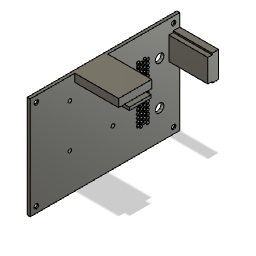
Main Pi Lid v6 (Autodesk Fusion 360 design; units mm, degrees)
Autodesk Fusion 360 part; units mm, degrees
sketch "Sketch1" plane through (0, 0, 0) normal (1, 0, 0) x (0, 0, -1)
  line L0 (-52, 35.5) -> (52, 35.5)
  line L1 (52, 35.5) -> (52, -35.5)
  line L2 (52, -35.5) -> (-52, -35.5)
  line L3 (-52, -35.5) -> (-52, 35.5)
  line L4 (-52, 35.5) -> (52, -35.5) construction
  line L5 (52, 35.5) -> (-52, -35.5) construction
  circle A0 centre (-47.75, 31.25) radius 1.55
  circle A1 centre (47.75, 31.25) radius 1.55
  circle A2 centre (47.75, -31.25) radius 1.55
  circle A3 centre (-47.75, -31.25) radius 1.55
  line L6 (20.5, 35.5) -> (-39.5, 35.5)
  line L7 (-39.5, 35.5) -> (-39.5, -24.5)
  line L8 (-39.5, -24.5) -> (20.5, -24.5)
  line L9 (20.5, -24.5) -> (20.5, 35.5)
  line L10 (20.5, 35.5) -> (-39.5, -24.5) construction
  line L11 (-39.5, 35.5) -> (20.5, -24.5) construction
  circle A4 centre (5.5, 20.5) radius 1.25
  circle A5 centre (-24.5, 20.5) radius 1.25
  circle A6 centre (-24.5, -9.5) radius 1.25
  circle A7 centre (5.5, -9.5) radius 1.25
  circle A8 centre (38, 15) radius 3
  circle A9 centre (38, -15) radius 3
  line L12 (22.4227, 20.645) -> (21.8453, 19.645)
  line L13 (21.8453, 19.645) -> (22.4227, 18.645)
  line L14 (22.4227, 18.645) -> (23.5774, 18.645)
  line L15 (23.5774, 18.645) -> (24.1547, 19.645)
  line L16 (24.1547, 19.645) -> (23.5774, 20.645)
  line L17 (23.5774, 20.645) -> (22.4227, 20.645)
  line L18 (24.653, 19.3561) -> (24.0756, 18.3561)
  line L19 (24.0756, 18.3561) -> (24.653, 17.3561)
  line L20 (24.653, 17.3561) -> (25.8077, 17.3561)
  line L21 (25.8077, 17.3561) -> (26.385, 18.3561)
  line L22 (26.385, 18.3561) -> (25.8077, 19.3561)
  line L23 (25.8077, 19.3561) -> (24.653, 19.3561)
  line L24 (30.3077, 19.3561) -> (29.153, 19.3561)
  line L25 (26.3453, 19.645) -> (26.9227, 18.645)
  line L26 (26.9227, 18.645) -> (28.0774, 18.645)
  line L27 (29.153, 19.3561) -> (28.5756, 18.3561)
  line L28 (29.153, 17.3561) -> (30.3077, 17.3561)
  line L29 (30.3077, 17.3561) -> (30.885, 18.3561)
  line L30 (28.6547, 19.645) -> (28.0774, 20.645)
  line L31 (28.5756, 18.3561) -> (29.153, 17.3561)
  line L32 (28.0774, 20.645) -> (26.9227, 20.645)
  line L33 (30.885, 18.3561) -> (30.3077, 19.3561)
  line L34 (28.0774, 18.645) -> (28.6547, 19.645)
  line L35 (26.9227, 20.645) -> (26.3453, 19.645)
  line L36 (25.8077, 16.8228) -> (24.653, 16.8228)
  line L37 (21.8453, 17.1117) -> (22.4227, 16.1117)
  line L38 (22.4227, 16.1117) -> (23.5774, 16.1117)
  line L39 (24.653, 16.8228) -> (24.0756, 15.8228)
  line L40 (24.653, 14.8228) -> (25.8077, 14.8228)
  line L41 (25.8077, 14.8228) -> (26.385, 15.8228)
  line L42 (24.1547, 17.1117) -> (23.5774, 18.1117)
  line L43 (24.0756, 15.8228) -> (24.653, 14.8228)
  line L44 (23.5774, 18.1117) -> (22.4227, 18.1117)
  line L45 (26.385, 15.8228) -> (25.8077, 16.8228)
  line L46 (23.5774, 16.1117) -> (24.1547, 17.1117)
  line L47 (22.4227, 18.1117) -> (21.8453, 17.1117)
  line L48 (30.3077, 16.8228) -> (29.153, 16.8228)
  line L49 (26.3453, 17.1117) -> (26.9227, 16.1117)
  line L50 (26.9227, 16.1117) -> (28.0774, 16.1117)
  line L51 (29.153, 16.8228) -> (28.5756, 15.8228)
  line L52 (29.153, 14.8228) -> (30.3077, 14.8228)
  line L53 (30.3077, 14.8228) -> (30.885, 15.8228)
  line L54 (28.6547, 17.1117) -> (28.0774, 18.1117)
  line L55 (28.5756, 15.8228) -> (29.153, 14.8228)
  line L56 (28.0774, 18.1117) -> (26.9227, 18.1117)
  line L57 (30.885, 15.8228) -> (30.3077, 16.8228)
  line L58 (28.0774, 16.1117) -> (28.6547, 17.1117)
  line L59 (26.9227, 18.1117) -> (26.3453, 17.1117)
  line L60 (25.8077, 14.2895) -> (24.653, 14.2895)
  line L61 (21.8453, 14.5783) -> (22.4227, 13.5783)
  line L62 (22.4227, 13.5783) -> (23.5774, 13.5783)
  line L63 (24.653, 14.2895) -> (24.0756, 13.2895)
  line L64 (24.653, 12.2895) -> (25.8077, 12.2895)
  line L65 (25.8077, 12.2895) -> (26.385, 13.2895)
  line L66 (24.1547, 14.5783) -> (23.5774, 15.5783)
  line L67 (24.0756, 13.2895) -> (24.653, 12.2895)
  line L68 (23.5774, 15.5783) -> (22.4227, 15.5783)
  line L69 (26.385, 13.2895) -> (25.8077, 14.2895)
  line L70 (23.5774, 13.5783) -> (24.1547, 14.5783)
  line L71 (22.4227, 15.5783) -> (21.8453, 14.5783)
  line L72 (30.3077, 14.2895) -> (29.153, 14.2895)
  line L73 (26.3453, 14.5783) -> (26.9227, 13.5783)
  line L74 (26.9227, 13.5783) -> (28.0774, 13.5783)
  line L75 (29.153, 14.2895) -> (28.5756, 13.2895)
  line L76 (29.153, 12.2895) -> (30.3077, 12.2895)
  line L77 (30.3077, 12.2895) -> (30.885, 13.2895)
  line L78 (28.6547, 14.5783) -> (28.0774, 15.5783)
  line L79 (28.5756, 13.2895) -> (29.153, 12.2895)
  line L80 (28.0774, 15.5783) -> (26.9227, 15.5783)
  line L81 (30.885, 13.2895) -> (30.3077, 14.2895)
  line L82 (28.0774, 13.5783) -> (28.6547, 14.5783)
  line L83 (26.9227, 15.5783) -> (26.3453, 14.5783)
  line L84 (25.8077, 11.7561) -> (24.653, 11.7561)
  line L85 (21.8453, 12.045) -> (22.4227, 11.045)
  line L86 (22.4227, 11.045) -> (23.5774, 11.045)
  line L87 (24.653, 11.7561) -> (24.0756, 10.7561)
  line L88 (24.653, 9.7561) -> (25.8077, 9.7561)
  line L89 (25.8077, 9.7561) -> (26.385, 10.7561)
  line L90 (24.1547, 12.045) -> (23.5774, 13.045)
  line L91 (24.0756, 10.7561) -> (24.653, 9.7561)
  line L92 (23.5774, 13.045) -> (22.4227, 13.045)
  line L93 (26.385, 10.7561) -> (25.8077, 11.7561)
  line L94 (23.5774, 11.045) -> (24.1547, 12.045)
  line L95 (22.4227, 13.045) -> (21.8453, 12.045)
  line L96 (30.3077, 11.7561) -> (29.153, 11.7561)
  line L97 (26.3453, 12.045) -> (26.9227, 11.045)
  line L98 (26.9227, 11.045) -> (28.0774, 11.045)
  line L99 (29.153, 11.7561) -> (28.5756, 10.7561)
  line L100 (29.153, 9.7561) -> (30.3077, 9.7561)
  line L101 (30.3077, 9.7561) -> (30.885, 10.7561)
  line L102 (28.6547, 12.045) -> (28.0774, 13.045)
  line L103 (28.5756, 10.7561) -> (29.153, 9.7561)
  line L104 (28.0774, 13.045) -> (26.9227, 13.045)
  line L105 (30.885, 10.7561) -> (30.3077, 11.7561)
  line L106 (28.0774, 11.045) -> (28.6547, 12.045)
  line L107 (26.9227, 13.045) -> (26.3453, 12.045)
  line L108 (25.8077, 9.2228) -> (24.653, 9.2228)
  line L109 (21.8453, 9.5117) -> (22.4227, 8.5117)
  line L110 (22.4227, 8.5117) -> (23.5774, 8.5117)
  line L111 (24.653, 9.2228) -> (24.0756, 8.2228)
  line L112 (24.653, 7.2228) -> (25.8077, 7.2228)
  line L113 (25.8077, 7.2228) -> (26.385, 8.2228)
  line L114 (24.1547, 9.5117) -> (23.5774, 10.5117)
  line L115 (24.0756, 8.2228) -> (24.653, 7.2228)
  line L116 (23.5774, 10.5117) -> (22.4227, 10.5117)
  line L117 (26.385, 8.2228) -> (25.8077, 9.2228)
  line L118 (23.5774, 8.5117) -> (24.1547, 9.5117)
  line L119 (22.4227, 10.5117) -> (21.8453, 9.5117)
  line L120 (30.3077, 9.2228) -> (29.153, 9.2228)
  line L121 (26.3453, 9.5117) -> (26.9227, 8.5117)
  line L122 (26.9227, 8.5117) -> (28.0774, 8.5117)
  line L123 (29.153, 9.2228) -> (28.5756, 8.2228)
  line L124 (29.153, 7.2228) -> (30.3077, 7.2228)
  line L125 (30.3077, 7.2228) -> (30.885, 8.2228)
  line L126 (28.6547, 9.5117) -> (28.0774, 10.5117)
  line L127 (28.5756, 8.2228) -> (29.153, 7.2228)
  line L128 (28.0774, 10.5117) -> (26.9227, 10.5117)
  line L129 (30.885, 8.2228) -> (30.3077, 9.2228)
  line L130 (28.0774, 8.5117) -> (28.6547, 9.5117)
  line L131 (26.9227, 10.5117) -> (26.3453, 9.5117)
  line L132 (25.8077, 6.6895) -> (24.653, 6.6895)
  line L133 (21.8453, 6.9783) -> (22.4227, 5.9783)
  line L134 (22.4227, 5.9783) -> (23.5774, 5.9783)
  line L135 (24.653, 6.6895) -> (24.0756, 5.6895)
  line L136 (24.653, 4.6895) -> (25.8077, 4.6895)
  line L137 (25.8077, 4.6895) -> (26.385, 5.6895)
  line L138 (24.1547, 6.9783) -> (23.5774, 7.9783)
  line L139 (24.0756, 5.6895) -> (24.653, 4.6895)
  line L140 (23.5774, 7.9783) -> (22.4227, 7.9783)
  line L141 (26.385, 5.6895) -> (25.8077, 6.6895)
  line L142 (23.5774, 5.9783) -> (24.1547, 6.9783)
  line L143 (22.4227, 7.9783) -> (21.8453, 6.9783)
  line L144 (30.3077, 6.6895) -> (29.153, 6.6895)
  line L145 (26.3453, 6.9783) -> (26.9227, 5.9783)
  line L146 (26.9227, 5.9783) -> (28.0774, 5.9783)
  line L147 (29.153, 6.6895) -> (28.5756, 5.6895)
  line L148 (29.153, 4.6895) -> (30.3077, 4.6895)
  line L149 (30.3077, 4.6895) -> (30.885, 5.6895)
  line L150 (28.6547, 6.9783) -> (28.0774, 7.9783)
  line L151 (28.5756, 5.6895) -> (29.153, 4.6895)
  line L152 (28.0774, 7.9783) -> (26.9227, 7.9783)
  line L153 (30.885, 5.6895) -> (30.3077, 6.6895)
  line L154 (28.0774, 5.9783) -> (28.6547, 6.9783)
  line L155 (26.9227, 7.9783) -> (26.3453, 6.9783)
  line L156 (25.8077, 4.1561) -> (24.653, 4.1561)
  line L157 (21.8453, 4.445) -> (22.4227, 3.445)
  line L158 (22.4227, 3.445) -> (23.5774, 3.445)
  line L159 (24.653, 4.1561) -> (24.0756, 3.1561)
  line L160 (24.653, 2.1561) -> (25.8077, 2.1561)
  line L161 (25.8077, 2.1561) -> (26.385, 3.1561)
  line L162 (24.1547, 4.445) -> (23.5774, 5.445)
  line L163 (24.0756, 3.1561) -> (24.653, 2.1561)
  line L164 (23.5774, 5.445) -> (22.4227, 5.445)
  line L165 (26.385, 3.1561) -> (25.8077, 4.1561)
  line L166 (23.5774, 3.445) -> (24.1547, 4.445)
  line L167 (22.4227, 5.445) -> (21.8453, 4.445)
  line L168 (30.3077, 4.1561) -> (29.153, 4.1561)
  line L169 (26.3453, 4.445) -> (26.9227, 3.445)
  line L170 (26.9227, 3.445) -> (28.0774, 3.445)
  line L171 (29.153, 4.1561) -> (28.5756, 3.1561)
  line L172 (29.153, 2.1561) -> (30.3077, 2.1561)
  line L173 (30.3077, 2.1561) -> (30.885, 3.1561)
  line L174 (28.6547, 4.445) -> (28.0774, 5.445)
  line L175 (28.5756, 3.1561) -> (29.153, 2.1561)
  line L176 (28.0774, 5.445) -> (26.9227, 5.445)
  line L177 (30.885, 3.1561) -> (30.3077, 4.1561)
  line L178 (28.0774, 3.445) -> (28.6547, 4.445)
  line L179 (26.9227, 5.445) -> (26.3453, 4.445)
  line L180 (25.8077, 1.6228) -> (24.653, 1.6228)
  line L181 (21.8453, 1.9117) -> (22.4227, 0.9117)
  line L182 (22.4227, 0.9117) -> (23.5774, 0.9117)
  line L183 (24.653, 1.6228) -> (24.0756, 0.6228)
  line L184 (24.653, -0.3772) -> (25.8077, -0.3772)
  line L185 (25.8077, -0.3772) -> (26.385, 0.6228)
  line L186 (24.1547, 1.9117) -> (23.5774, 2.9117)
  line L187 (24.0756, 0.6228) -> (24.653, -0.3772)
  line L188 (23.5774, 2.9117) -> (22.4227, 2.9117)
  line L189 (26.385, 0.6228) -> (25.8077, 1.6228)
  line L190 (23.5774, 0.9117) -> (24.1547, 1.9117)
  line L191 (22.4227, 2.9117) -> (21.8453, 1.9117)
  line L192 (30.3077, 1.6228) -> (29.153, 1.6228)
  line L193 (26.3453, 1.9117) -> (26.9227, 0.9117)
  line L194 (26.9227, 0.9117) -> (28.0774, 0.9117)
  line L195 (29.153, 1.6228) -> (28.5756, 0.6228)
  line L196 (29.153, -0.3772) -> (30.3077, -0.3772)
  line L197 (30.3077, -0.3772) -> (30.885, 0.6228)
  line L198 (28.6547, 1.9117) -> (28.0774, 2.9117)
  line L199 (28.5756, 0.6228) -> (29.153, -0.3772)
  line L200 (28.0774, 2.9117) -> (26.9227, 2.9117)
  line L201 (30.885, 0.6228) -> (30.3077, 1.6228)
  line L202 (28.0774, 0.9117) -> (28.6547, 1.9117)
  line L203 (26.9227, 2.9117) -> (26.3453, 1.9117)
  line L204 (25.8077, -0.9105) -> (24.653, -0.9105)
  line L205 (21.8453, -0.6217) -> (22.4227, -1.6217)
  line L206 (22.4227, -1.6217) -> (23.5774, -1.6217)
  line L207 (24.653, -0.9105) -> (24.0756, -1.9105)
  line L208 (24.653, -2.9105) -> (25.8077, -2.9105)
  line L209 (25.8077, -2.9105) -> (26.385, -1.9105)
  line L210 (24.1547, -0.6217) -> (23.5774, 0.3783)
  line L211 (24.0756, -1.9105) -> (24.653, -2.9105)
  line L212 (23.5774, 0.3783) -> (22.4227, 0.3783)
  line L213 (26.385, -1.9105) -> (25.8077, -0.9105)
  line L214 (23.5774, -1.6217) -> (24.1547, -0.6217)
  line L215 (22.4227, 0.3783) -> (21.8453, -0.6217)
  line L216 (30.3077, -0.9105) -> (29.153, -0.9105)
  line L217 (26.3453, -0.6217) -> (26.9227, -1.6217)
  line L218 (26.9227, -1.6217) -> (28.0774, -1.6217)
  line L219 (29.153, -0.9105) -> (28.5756, -1.9105)
  line L220 (29.153, -2.9105) -> (30.3077, -2.9105)
  line L221 (30.3077, -2.9105) -> (30.885, -1.9105)
  line L222 (28.6547, -0.6217) -> (28.0774, 0.3783)
  line L223 (28.5756, -1.9105) -> (29.153, -2.9105)
  line L224 (28.0774, 0.3783) -> (26.9227, 0.3783)
  line L225 (30.885, -1.9105) -> (30.3077, -0.9105)
  line L226 (28.0774, -1.6217) -> (28.6547, -0.6217)
  line L227 (26.9227, 0.3783) -> (26.3453, -0.6217)
  line L228 (25.8077, -3.4439) -> (24.653, -3.4439)
  line L229 (21.8453, -3.155) -> (22.4227, -4.155)
  line L230 (22.4227, -4.155) -> (23.5774, -4.155)
  line L231 (24.653, -3.4439) -> (24.0756, -4.4439)
  line L232 (24.653, -5.4439) -> (25.8077, -5.4439)
  line L233 (25.8077, -5.4439) -> (26.385, -4.4439)
  line L234 (24.1547, -3.155) -> (23.5774, -2.155)
  line L235 (24.0756, -4.4439) -> (24.653, -5.4439)
  line L236 (23.5774, -2.155) -> (22.4227, -2.155)
  line L237 (26.385, -4.4439) -> (25.8077, -3.4439)
  line L238 (23.5774, -4.155) -> (24.1547, -3.155)
  line L239 (22.4227, -2.155) -> (21.8453, -3.155)
  line L240 (30.3077, -3.4439) -> (29.153, -3.4439)
  line L241 (26.3453, -3.155) -> (26.9227, -4.155)
  line L242 (26.9227, -4.155) -> (28.0774, -4.155)
  line L243 (29.153, -3.4439) -> (28.5756, -4.4439)
  line L244 (29.153, -5.4439) -> (30.3077, -5.4439)
  line L245 (30.3077, -5.4439) -> (30.885, -4.4439)
  line L246 (28.6547, -3.155) -> (28.0774, -2.155)
  line L247 (28.5756, -4.4439) -> (29.153, -5.4439)
  line L248 (28.0774, -2.155) -> (26.9227, -2.155)
  line L249 (30.885, -4.4439) -> (30.3077, -3.4439)
  line L250 (28.0774, -4.155) -> (28.6547, -3.155)
  line L251 (26.9227, -2.155) -> (26.3453, -3.155)
  line L252 (25.8077, -5.9772) -> (24.653, -5.9772)
  line L253 (21.8453, -5.6883) -> (22.4227, -6.6883)
  line L254 (22.4227, -6.6883) -> (23.5774, -6.6883)
  line L255 (24.653, -5.9772) -> (24.0756, -6.9772)
  line L256 (24.653, -7.9772) -> (25.8077, -7.9772)
  line L257 (25.8077, -7.9772) -> (26.385, -6.9772)
  line L258 (24.1547, -5.6883) -> (23.5774, -4.6883)
  line L259 (24.0756, -6.9772) -> (24.653, -7.9772)
  line L260 (23.5774, -4.6883) -> (22.4227, -4.6883)
  line L261 (26.385, -6.9772) -> (25.8077, -5.9772)
  line L262 (23.5774, -6.6883) -> (24.1547, -5.6883)
  line L263 (22.4227, -4.6883) -> (21.8453, -5.6883)
  line L264 (30.3077, -5.9772) -> (29.153, -5.9772)
  line L265 (26.3453, -5.6883) -> (26.9227, -6.6883)
  line L266 (26.9227, -6.6883) -> (28.0774, -6.6883)
  line L267 (29.153, -5.9772) -> (28.5756, -6.9772)
  line L268 (29.153, -7.9772) -> (30.3077, -7.9772)
  line L269 (30.3077, -7.9772) -> (30.885, -6.9772)
  line L270 (28.6547, -5.6883) -> (28.0774, -4.6883)
  line L271 (28.5756, -6.9772) -> (29.153, -7.9772)
  line L272 (28.0774, -4.6883) -> (26.9227, -4.6883)
  line L273 (30.885, -6.9772) -> (30.3077, -5.9772)
  line L274 (28.0774, -6.6883) -> (28.6547, -5.6883)
  line L275 (26.9227, -4.6883) -> (26.3453, -5.6883)
  line L276 (25.8077, -8.5105) -> (24.653, -8.5105)
  line L277 (21.8453, -8.2217) -> (22.4227, -9.2217)
  line L278 (22.4227, -9.2217) -> (23.5774, -9.2217)
  line L279 (24.653, -8.5105) -> (24.0756, -9.5105)
  line L280 (24.653, -10.5105) -> (25.8077, -10.5105)
  line L281 (25.8077, -10.5105) -> (26.385, -9.5105)
  line L282 (24.1547, -8.2217) -> (23.5774, -7.2217)
  line L283 (24.0756, -9.5105) -> (24.653, -10.5105)
  line L284 (23.5774, -7.2217) -> (22.4227, -7.2217)
  line L285 (26.385, -9.5105) -> (25.8077, -8.5105)
  line L286 (23.5774, -9.2217) -> (24.1547, -8.2217)
  line L287 (22.4227, -7.2217) -> (21.8453, -8.2217)
  line L288 (30.3077, -8.5105) -> (29.153, -8.5105)
  line L289 (26.3453, -8.2217) -> (26.9227, -9.2217)
  line L290 (26.9227, -9.2217) -> (28.0774, -9.2217)
  line L291 (29.153, -8.5105) -> (28.5756, -9.5105)
  line L292 (29.153, -10.5105) -> (30.3077, -10.5105)
  line L293 (30.3077, -10.5105) -> (30.885, -9.5105)
  line L294 (28.6547, -8.2217) -> (28.0774, -7.2217)
  line L295 (28.5756, -9.5105) -> (29.153, -10.5105)
  line L296 (28.0774, -7.2217) -> (26.9227, -7.2217)
  line L297 (30.885, -9.5105) -> (30.3077, -8.5105)
  line L298 (28.0774, -9.2217) -> (28.6547, -8.2217)
  line L299 (26.9227, -7.2217) -> (26.3453, -8.2217)
  line L300 (25.8077, -11.0439) -> (24.653, -11.0439)
  line L301 (21.8453, -10.755) -> (22.4227, -11.755)
  line L302 (22.4227, -11.755) -> (23.5774, -11.755)
  line L303 (24.653, -11.0439) -> (24.0756, -12.0439)
  line L304 (24.653, -13.0439) -> (25.8077, -13.0439)
  line L305 (25.8077, -13.0439) -> (26.385, -12.0439)
  line L306 (24.1547, -10.755) -> (23.5774, -9.755)
  line L307 (24.0756, -12.0439) -> (24.653, -13.0439)
  line L308 (23.5774, -9.755) -> (22.4227, -9.755)
  line L309 (26.385, -12.0439) -> (25.8077, -11.0439)
  line L310 (23.5774, -11.755) -> (24.1547, -10.755)
  line L311 (22.4227, -9.755) -> (21.8453, -10.755)
  line L312 (30.3077, -11.0439) -> (29.153, -11.0439)
  line L313 (26.3453, -10.755) -> (26.9227, -11.755)
  line L314 (26.9227, -11.755) -> (28.0774, -11.755)
  line L315 (29.153, -11.0439) -> (28.5756, -12.0439)
  line L316 (29.153, -13.0439) -> (30.3077, -13.0439)
  line L317 (30.3077, -13.0439) -> (30.885, -12.0439)
  line L318 (28.6547, -10.755) -> (28.0774, -9.755)
  line L319 (28.5756, -12.0439) -> (29.153, -13.0439)
  line L320 (28.0774, -9.755) -> (26.9227, -9.755)
  line L321 (30.885, -12.0439) -> (30.3077, -11.0439)
  line L322 (28.0774, -11.755) -> (28.6547, -10.755)
  line L323 (26.9227, -9.755) -> (26.3453, -10.755)
  line L324 (25.8077, -13.5772) -> (24.653, -13.5772)
  line L325 (21.8453, -13.2883) -> (22.4227, -14.2883)
  line L326 (22.4227, -14.2883) -> (23.5774, -14.2883)
  line L327 (24.653, -13.5772) -> (24.0756, -14.5772)
  line L328 (24.653, -15.5772) -> (25.8077, -15.5772)
  line L329 (25.8077, -15.5772) -> (26.385, -14.5772)
  line L330 (24.1547, -13.2883) -> (23.5774, -12.2883)
  line L331 (24.0756, -14.5772) -> (24.653, -15.5772)
  line L332 (23.5774, -12.2883) -> (22.4227, -12.2883)
  line L333 (26.385, -14.5772) -> (25.8077, -13.5772)
  line L334 (23.5774, -14.2883) -> (24.1547, -13.2883)
  line L335 (22.4227, -12.2883) -> (21.8453, -13.2883)
  line L336 (30.3077, -13.5772) -> (29.153, -13.5772)
  line L337 (26.3453, -13.2883) -> (26.9227, -14.2883)
  line L338 (26.9227, -14.2883) -> (28.0774, -14.2883)
  line L339 (29.153, -13.5772) -> (28.5756, -14.5772)
  line L340 (29.153, -15.5772) -> (30.3077, -15.5772)
  line L341 (30.3077, -15.5772) -> (30.885, -14.5772)
  line L342 (28.6547, -13.2883) -> (28.0774, -12.2883)
  line L343 (28.5756, -14.5772) -> (29.153, -15.5772)
  line L344 (28.0774, -12.2883) -> (26.9227, -12.2883)
  line L345 (30.885, -14.5772) -> (30.3077, -13.5772)
  line L346 (28.0774, -14.2883) -> (28.6547, -13.2883)
  line L347 (26.9227, -12.2883) -> (26.3453, -13.2883)
  line L348 (25.8077, -16.1105) -> (24.653, -16.1105)
  line L349 (21.8453, -15.8217) -> (22.4227, -16.8217)
  line L350 (22.4227, -16.8217) -> (23.5774, -16.8217)
  line L351 (24.653, -16.1105) -> (24.0756, -17.1105)
  line L352 (24.653, -18.1105) -> (25.8077, -18.1105)
  line L353 (25.8077, -18.1105) -> (26.385, -17.1105)
  line L354 (24.1547, -15.8217) -> (23.5774, -14.8217)
  line L355 (24.0756, -17.1105) -> (24.653, -18.1105)
  line L356 (23.5774, -14.8217) -> (22.4227, -14.8217)
  line L357 (26.385, -17.1105) -> (25.8077, -16.1105)
  line L358 (23.5774, -16.8217) -> (24.1547, -15.8217)
  line L359 (22.4227, -14.8217) -> (21.8453, -15.8217)
  line L360 (30.3077, -16.1105) -> (29.153, -16.1105)
  line L361 (26.3453, -15.8217) -> (26.9227, -16.8217)
  line L362 (26.9227, -16.8217) -> (28.0774, -16.8217)
  line L363 (29.153, -16.1105) -> (28.5756, -17.1105)
  line L364 (29.153, -18.1105) -> (30.3077, -18.1105)
  line L365 (30.3077, -18.1105) -> (30.885, -17.1105)
  line L366 (28.6547, -15.8217) -> (28.0774, -14.8217)
  line L367 (28.5756, -17.1105) -> (29.153, -18.1105)
  line L368 (28.0774, -14.8217) -> (26.9227, -14.8217)
  line L369 (30.885, -17.1105) -> (30.3077, -16.1105)
  line L370 (28.0774, -16.8217) -> (28.6547, -15.8217)
  line L371 (26.9227, -14.8217) -> (26.3453, -15.8217)
  line L372 (25.8077, -18.6439) -> (24.653, -18.6439)
  line L373 (21.8453, -18.355) -> (22.4227, -19.355)
  line L374 (22.4227, -19.355) -> (23.5774, -19.355)
  line L375 (24.653, -18.6439) -> (24.0756, -19.6439)
  line L376 (24.653, -20.6439) -> (25.8077, -20.6439)
  line L377 (25.8077, -20.6439) -> (26.385, -19.6439)
  line L378 (24.1547, -18.355) -> (23.5774, -17.355)
  line L379 (24.0756, -19.6439) -> (24.653, -20.6439)
  line L380 (23.5774, -17.355) -> (22.4227, -17.355)
  line L381 (26.385, -19.6439) -> (25.8077, -18.6439)
  line L382 (23.5774, -19.355) -> (24.1547, -18.355)
  line L383 (22.4227, -17.355) -> (21.8453, -18.355)
  line L384 (30.3077, -18.6439) -> (29.153, -18.6439)
  line L385 (26.3453, -18.355) -> (26.9227, -19.355)
  line L386 (26.9227, -19.355) -> (28.0774, -19.355)
  line L387 (29.153, -18.6439) -> (28.5756, -19.6439)
  line L388 (29.153, -20.6439) -> (30.3077, -20.6439)
  line L389 (30.3077, -20.6439) -> (30.885, -19.6439)
  line L390 (28.6547, -18.355) -> (28.0774, -17.355)
  line L391 (28.5756, -19.6439) -> (29.153, -20.6439)
  line L392 (28.0774, -17.355) -> (26.9227, -17.355)
  line L393 (30.885, -19.6439) -> (30.3077, -18.6439)
  line L394 (28.0774, -19.355) -> (28.6547, -18.355)
  line L395 (26.9227, -17.355) -> (26.3453, -18.355)
  point P0 (-9.5, 5.5)
  point P1 (23, 19.645)
  point P2 (25.2303, 18.3561)
  point P3 (29.7303, 18.3561)
  point P4 (27.5, 19.645)
  point P5 (25.2303, 15.8228)
  point P6 (23, 17.1117)
  point P7 (29.7303, 15.8228)
  point P8 (27.5, 17.1117)
  point P9 (25.2303, 13.2895)
  point P10 (23, 14.5783)
  point P11 (29.7303, 13.2895)
  point P12 (27.5, 14.5783)
  point P13 (25.2303, 10.7561)
  point P14 (23, 12.045)
  point P15 (29.7303, 10.7561)
  point P16 (27.5, 12.045)
  point P17 (25.2303, 8.2228)
  point P18 (23, 9.5117)
  point P19 (29.7303, 8.2228)
  point P20 (27.5, 9.5117)
  point P21 (25.2303, 5.6895)
  point P22 (23, 6.9783)
  point P23 (29.7303, 5.6895)
  point P24 (27.5, 6.9783)
  point P25 (25.2303, 3.1561)
  point P26 (23, 4.445)
  point P27 (29.7303, 3.1561)
  point P28 (27.5, 4.445)
  point P29 (25.2303, 0.6228)
  point P30 (23, 1.9117)
  point P31 (29.7303, 0.6228)
  point P32 (27.5, 1.9117)
  point P33 (25.2303, -1.9105)
  point P34 (23, -0.6217)
  point P35 (29.7303, -1.9105)
  point P36 (27.5, -0.6217)
  point P37 (25.2303, -4.4439)
  point P38 (23, -3.155)
  point P39 (29.7303, -4.4439)
  point P40 (27.5, -3.155)
  point P41 (25.2303, -6.9772)
  point P42 (23, -5.6883)
  point P43 (29.7303, -6.9772)
  point P44 (27.5, -5.6883)
  point P45 (25.2303, -9.5105)
  point P46 (23, -8.2217)
  point P47 (29.7303, -9.5105)
  point P48 (27.5, -8.2217)
  point P49 (25.2303, -12.0439)
  point P50 (23, -10.755)
  point P51 (29.7303, -12.0439)
  point P52 (27.5, -10.755)
  point P53 (25.2303, -14.5772)
  point P54 (23, -13.2883)
  point P55 (29.7303, -14.5772)
  point P56 (27.5, -13.2883)
  point P57 (25.2303, -17.1105)
  point P58 (23, -15.8217)
  point P59 (29.7303, -17.1105)
  point P60 (27.5, -15.8217)
  point P61 (25.2303, -19.6439)
  point P62 (23, -18.355)
  point P63 (29.7303, -19.6439)
  point P64 (27.5, -18.355)
  dimension "d1" = 104
  dimension "d2" = 71
  dimension "d3" = 3.1
  dimension "d4" = 3.1
  dimension "d5" = 3.1
  dimension "d6" = 3.1
  dimension "d7" = 4.25
  dimension "d8" = 4.25
  dimension "d9" = 4.25
  dimension "d10" = 4.25
  dimension "d11" = 4.25
  dimension "d12" = 4.25
  dimension "d13" = 4.25
  dimension "d14" = 4.25
  dimension "d27" = 60
  dimension "d28" = 60
  dimension "d29" = 2.5
  dimension "d30" = 2.5
  dimension "d31" = 2.5
  dimension "d32" = 2.5
  dimension "d33" = 15
  dimension "d34" = 15
  dimension "d35" = 15
  dimension "d36" = 15
  dimension "d37" = 11
  dimension "d39" = 6
  dimension "d40" = 6
  dimension "d62" = 12.5
  dimension "d63" = 14
  dimension "d64" = 14
  dimension "d65" = 14.855
  dimension "d71" = 4.5
  dimension "d72" = -38
  dimension "d74" = 1
  dimension "d75" = 1
  dimension "d76" = 1.2889
  constraint horizontal L0
  constraint perpendicular L0 L1
  constraint parallel L0 L2
  constraint parallel L1 L3
  constraint coincident L4 origin
  constraint coincident L5 origin
  constraint horizontal L6
  constraint perpendicular L6 L7
  constraint parallel L6 L8
  constraint parallel L7 L9
  constraint coincident L10 P0
  constraint coincident L11 P0
  constraint coincident L10 A4.centre
  constraint coincident L11 A5.centre
  constraint coincident L10 A6.centre
  constraint coincident L11 A7.centre
  measures "d1" distance of L1.end L2.end
  measures "d2" distance of L0.end L1.end
  measures "d3" diameter of A0
  measures "d4" diameter of A1
  measures "d5" diameter of A2
  measures "d6" diameter of A3
  measures "d7" distance of L3 A0.centre
  measures "d8" distance of L0 A0.centre
  measures "d9" distance of L3 A3.centre
  measures "d10" distance of L2 A3.centre
  measures "d11" distance of L1 A1.centre
  measures "d12" distance of L0 A1.centre
  measures "d13" distance of L1 A2.centre
  measures "d14" distance of L2 A2.centre
  measures "d27" distance of L7.end L8.end
  measures "d28" distance of L6.end L7.end
  measures "d29" diameter of A4
  measures "d30" diameter of A5
  measures "d31" diameter of A6
  measures "d32" diameter of A7
  measures "d33" distance of L9 A7.centre
  measures "d34" distance of L7 A6.centre
  measures "d35" distance of L7 A5.centre
  measures "d36" distance of L9 A4.centre
  measures "d37" distance of L2 L8
  measures "d39" diameter of A8
  measures "d40" diameter of A9
  measures "d62" distance of L3 L7
  measures "d63" distance of L1 A8.centre
  measures "d64" distance of L1 A9.centre
  measures "d65" distance of L0 L12.start
  measures "d74" distance of P1 L16
  measures "d75" distance of P2 L22
  measures "d76" distance of L23 L32
extrude "Extrude1" add sketch "Sketch1" along normal blind 2
chamfer "Chamfer1" distance 1.25 angle 45 4 edges at (0, -30.6895, 49.1951) (0, -30.6895, -46.3049) (0, 31.8105, -46.3049) (0, 31.8105, 49.1951)
sketch "Sketch2" plane through (2, 0, 0) normal (1, 0, 0) x (0, 0, -1)
  circle A0 centre (-24.5, -9.5) radius 1.25
  circle A1 centre (47.75, 31.25) radius 1.55
  circle A2 centre (5.5, 20.5) radius 1.25
  circle A3 centre (-24.5, 20.5) radius 1.25
  circle A4 centre (5.5, -9.5) radius 1.25
  circle A5 centre (38, -15) radius 3
  circle A6 centre (47.75, -31.25) radius 1.55
  circle A7 centre (-47.75, -31.25) radius 1.55
  circle A8 centre (38, 15) radius 3
  circle A9 centre (-47.75, 31.25) radius 1.55
  line L0 (-52, -35.5) -> (52, -35.5)
  line L1 (52, -35.5) -> (52, 35.5)
  line L2 (52, 35.5) -> (-52, 35.5)
  line L3 (-52, 35.5) -> (-52, -35.5)
  line L4 (-21, 35.5) -> (2, 35.5)
  line L5 (2, 35.5) -> (2, 30)
  line L6 (2, 30) -> (-21, 30)
  line L7 (-21, 30) -> (-21, 35.5)
  line L8 (-17, 30) -> (-2, 30)
  line L9 (-2, 30) -> (-2, 28)
  line L10 (-2, 28) -> (-17, 28)
  line L11 (-17, 28) -> (-17, 30)
  line L12 (52, 26.75) -> (47.5, 26.75)
  line L13 (47.5, 26.75) -> (47.5, 8.75)
  line L14 (47.5, 8.75) -> (52, 8.75)
  line L15 (52, 8.75) -> (52, 26.75)
  line L16 (47.5, 25.75) -> (44.5, 25.75)
  line L17 (44.5, 25.75) -> (44.5, 9.75)
  line L18 (44.5, 9.75) -> (47.5, 9.75)
  line L19 (47.5, 9.75) -> (47.5, 25.75)
  line L20 (25.8077, 9.2228) -> (26.385, 8.2228)
  line L21 (26.385, 8.2228) -> (25.8077, 7.2228)
  line L22 (25.8077, 7.2228) -> (24.653, 7.2228)
  line L23 (24.653, 7.2228) -> (24.0756, 8.2228)
  line L24 (24.0756, 8.2228) -> (24.653, 9.2228)
  line L25 (24.653, 9.2228) -> (25.8077, 9.2228)
  line L26 (21.8453, -3.155) -> (22.4227, -2.155)
  line L27 (22.4227, -2.155) -> (23.5774, -2.155)
  line L28 (23.5774, -2.155) -> (24.1547, -3.155)
  line L29 (24.1547, -3.155) -> (23.5774, -4.155)
  line L30 (23.5774, -4.155) -> (22.4227, -4.155)
  line L31 (22.4227, -4.155) -> (21.8453, -3.155)
  line L32 (26.3453, -3.155) -> (26.9227, -2.155)
  line L33 (26.9227, -2.155) -> (28.0774, -2.155)
  line L34 (28.0774, -2.155) -> (28.6547, -3.155)
  line L35 (28.6547, -3.155) -> (28.0774, -4.155)
  line L36 (28.0774, -4.155) -> (26.9227, -4.155)
  line L37 (26.9227, -4.155) -> (26.3453, -3.155)
  line L38 (25.8077, -5.9772) -> (26.385, -6.9772)
  line L39 (26.385, -6.9772) -> (25.8077, -7.9772)
  line L40 (25.8077, -7.9772) -> (24.653, -7.9772)
  line L41 (24.653, -7.9772) -> (24.0756, -6.9772)
  line L42 (24.0756, -6.9772) -> (24.653, -5.9772)
  line L43 (24.653, -5.9772) -> (25.8077, -5.9772)
  line L44 (21.8453, -15.8217) -> (22.4227, -14.8217)
  line L45 (22.4227, -14.8217) -> (23.5774, -14.8217)
  line L46 (23.5774, -14.8217) -> (24.1547, -15.8217)
  line L47 (24.1547, -15.8217) -> (23.5774, -16.8217)
  line L48 (23.5774, -16.8217) -> (22.4227, -16.8217)
  line L49 (22.4227, -16.8217) -> (21.8453, -15.8217)
  line L50 (26.3453, 19.645) -> (26.9227, 20.645)
  line L51 (26.9227, 20.645) -> (28.0774, 20.645)
  line L52 (28.0774, 20.645) -> (28.6547, 19.645)
  line L53 (28.6547, 19.645) -> (28.0774, 18.645)
  line L54 (28.0774, 18.645) -> (26.9227, 18.645)
  line L55 (26.9227, 18.645) -> (26.3453, 19.645)
  line L56 (21.8453, 17.1117) -> (22.4227, 18.1117)
  line L57 (22.4227, 18.1117) -> (23.5774, 18.1117)
  line L58 (23.5774, 18.1117) -> (24.1547, 17.1117)
  line L59 (24.1547, 17.1117) -> (23.5774, 16.1117)
  line L60 (23.5774, 16.1117) -> (22.4227, 16.1117)
  line L61 (22.4227, 16.1117) -> (21.8453, 17.1117)
  line L62 (30.3077, -18.6439) -> (30.885, -19.6439)
  line L63 (30.885, -19.6439) -> (30.3077, -20.6439)
  line L64 (30.3077, -20.6439) -> (29.153, -20.6439)
  line L65 (29.153, -20.6439) -> (28.5756, -19.6439)
  line L66 (28.5756, -19.6439) -> (29.153, -18.6439)
  line L67 (29.153, -18.6439) -> (30.3077, -18.6439)
  line L68 (26.3453, 12.045) -> (26.9227, 13.045)
  line L69 (26.9227, 13.045) -> (28.0774, 13.045)
  line L70 (28.0774, 13.045) -> (28.6547, 12.045)
  line L71 (28.6547, 12.045) -> (28.0774, 11.045)
  line L72 (28.0774, 11.045) -> (26.9227, 11.045)
  line L73 (26.9227, 11.045) -> (26.3453, 12.045)
  line L74 (25.8077, -11.0439) -> (26.385, -12.0439)
  line L75 (26.385, -12.0439) -> (25.8077, -13.0439)
  line L76 (25.8077, -13.0439) -> (24.653, -13.0439)
  line L77 (24.653, -13.0439) -> (24.0756, -12.0439)
  line L78 (24.0756, -12.0439) -> (24.653, -11.0439)
  line L79 (24.653, -11.0439) -> (25.8077, -11.0439)
  line L80 (26.3453, 4.445) -> (26.9227, 5.445)
  line L81 (26.9227, 5.445) -> (28.0774, 5.445)
  line L82 (28.0774, 5.445) -> (28.6547, 4.445)
  line L83 (28.6547, 4.445) -> (28.0774, 3.445)
  line L84 (28.0774, 3.445) -> (26.9227, 3.445)
  line L85 (26.9227, 3.445) -> (26.3453, 4.445)
  line L86 (25.8077, 1.6228) -> (26.385, 0.6228)
  line L87 (26.385, 0.6228) -> (25.8077, -0.3772)
  line L88 (25.8077, -0.3772) -> (24.653, -0.3772)
  line L89 (24.653, -0.3772) -> (24.0756, 0.6228)
  line L90 (24.0756, 0.6228) -> (24.653, 1.6228)
  line L91 (24.653, 1.6228) -> (25.8077, 1.6228)
  line L92 (30.3077, 4.1561) -> (30.885, 3.1561)
  line L93 (30.885, 3.1561) -> (30.3077, 2.1561)
  line L94 (30.3077, 2.1561) -> (29.153, 2.1561)
  line L95 (29.153, 2.1561) -> (28.5756, 3.1561)
  line L96 (28.5756, 3.1561) -> (29.153, 4.1561)
  line L97 (29.153, 4.1561) -> (30.3077, 4.1561)
  line L98 (30.3077, 1.6228) -> (30.885, 0.6228)
  line L99 (30.885, 0.6228) -> (30.3077, -0.3772)
  line L100 (30.3077, -0.3772) -> (29.153, -0.3772)
  line L101 (29.153, -0.3772) -> (28.5756, 0.6228)
  line L102 (28.5756, 0.6228) -> (29.153, 1.6228)
  line L103 (29.153, 1.6228) -> (30.3077, 1.6228)
  line L104 (22.4227, 20.645) -> (23.5774, 20.645)
  line L105 (23.5774, 20.645) -> (24.1547, 19.645)
  line L106 (24.1547, 19.645) -> (23.5774, 18.645)
  line L107 (23.5774, 18.645) -> (22.4227, 18.645)
  line L108 (22.4227, 18.645) -> (21.8453, 19.645)
  line L109 (21.8453, 19.645) -> (22.4227, 20.645)
  line L110 (30.3077, 19.3561) -> (30.885, 18.3561)
  line L111 (30.885, 18.3561) -> (30.3077, 17.3561)
  line L112 (30.3077, 17.3561) -> (29.153, 17.3561)
  line L113 (29.153, 17.3561) -> (28.5756, 18.3561)
  line L114 (28.5756, 18.3561) -> (29.153, 19.3561)
  line L115 (29.153, 19.3561) -> (30.3077, 19.3561)
  line L116 (25.8077, -0.9105) -> (26.385, -1.9105)
  line L117 (26.385, -1.9105) -> (25.8077, -2.9105)
  line L118 (25.8077, -2.9105) -> (24.653, -2.9105)
  line L119 (24.653, -2.9105) -> (24.0756, -1.9105)
  line L120 (24.0756, -1.9105) -> (24.653, -0.9105)
  line L121 (24.653, -0.9105) -> (25.8077, -0.9105)
  line L122 (21.8453, 1.9117) -> (22.4227, 2.9117)
  line L123 (22.4227, 2.9117) -> (23.5774, 2.9117)
  line L124 (23.5774, 2.9117) -> (24.1547, 1.9117)
  line L125 (24.1547, 1.9117) -> (23.5774, 0.9117)
  line L126 (23.5774, 0.9117) -> (22.4227, 0.9117)
  line L127 (22.4227, 0.9117) -> (21.8453, 1.9117)
  line L128 (21.8453, -0.6217) -> (22.4227, 0.3783)
  line L129 (22.4227, 0.3783) -> (23.5774, 0.3783)
  line L130 (23.5774, 0.3783) -> (24.1547, -0.6217)
  line L131 (24.1547, -0.6217) -> (23.5774, -1.6217)
  line L132 (23.5774, -1.6217) -> (22.4227, -1.6217)
  line L133 (22.4227, -1.6217) -> (21.8453, -0.6217)
  line L134 (26.3453, -0.6217) -> (26.9227, 0.3783)
  line L135 (26.9227, 0.3783) -> (28.0774, 0.3783)
  line L136 (28.0774, 0.3783) -> (28.6547, -0.6217)
  line L137 (28.6547, -0.6217) -> (28.0774, -1.6217)
  line L138 (28.0774, -1.6217) -> (26.9227, -1.6217)
  line L139 (26.9227, -1.6217) -> (26.3453, -0.6217)
  line L140 (25.8077, 16.8228) -> (26.385, 15.8228)
  line L141 (26.385, 15.8228) -> (25.8077, 14.8228)
  line L142 (25.8077, 14.8228) -> (24.653, 14.8228)
  line L143 (24.653, 14.8228) -> (24.0756, 15.8228)
  line L144 (24.0756, 15.8228) -> (24.653, 16.8228)
  line L145 (24.653, 16.8228) -> (25.8077, 16.8228)
  line L146 (25.8077, -3.4439) -> (26.385, -4.4439)
  line L147 (26.385, -4.4439) -> (25.8077, -5.4439)
  line L148 (25.8077, -5.4439) -> (24.653, -5.4439)
  line L149 (24.653, -5.4439) -> (24.0756, -4.4439)
  line L150 (24.0756, -4.4439) -> (24.653, -3.4439)
  line L151 (24.653, -3.4439) -> (25.8077, -3.4439)
  line L152 (26.3453, 1.9117) -> (26.9227, 2.9117)
  line L153 (26.9227, 2.9117) -> (28.0774, 2.9117)
  line L154 (28.0774, 2.9117) -> (28.6547, 1.9117)
  line L155 (28.6547, 1.9117) -> (28.0774, 0.9117)
  line L156 (28.0774, 0.9117) -> (26.9227, 0.9117)
  line L157 (26.9227, 0.9117) -> (26.3453, 1.9117)
  line L158 (30.3077, -0.9105) -> (30.885, -1.9105)
  line L159 (30.885, -1.9105) -> (30.3077, -2.9105)
  line L160 (30.3077, -2.9105) -> (29.153, -2.9105)
  line L161 (29.153, -2.9105) -> (28.5756, -1.9105)
  line L162 (28.5756, -1.9105) -> (29.153, -0.9105)
  line L163 (29.153, -0.9105) -> (30.3077, -0.9105)
  line L164 (30.3077, 6.6895) -> (30.885, 5.6895)
  line L165 (30.885, 5.6895) -> (30.3077, 4.6895)
  line L166 (30.3077, 4.6895) -> (29.153, 4.6895)
  line L167 (29.153, 4.6895) -> (28.5756, 5.6895)
  line L168 (28.5756, 5.6895) -> (29.153, 6.6895)
  line L169 (29.153, 6.6895) -> (30.3077, 6.6895)
  line L170 (21.8453, 6.9783) -> (22.4227, 7.9783)
  line L171 (22.4227, 7.9783) -> (23.5774, 7.9783)
  line L172 (23.5774, 7.9783) -> (24.1547, 6.9783)
  line L173 (24.1547, 6.9783) -> (23.5774, 5.9783)
  line L174 (23.5774, 5.9783) -> (22.4227, 5.9783)
  line L175 (22.4227, 5.9783) -> (21.8453, 6.9783)
  line L176 (26.3453, 6.9783) -> (26.9227, 7.9783)
  line L177 (26.9227, 7.9783) -> (28.0774, 7.9783)
  line L178 (28.0774, 7.9783) -> (28.6547, 6.9783)
  line L179 (28.6547, 6.9783) -> (28.0774, 5.9783)
  line L180 (28.0774, 5.9783) -> (26.9227, 5.9783)
  line L181 (26.9227, 5.9783) -> (26.3453, 6.9783)
  line L182 (24.653, 19.3561) -> (25.8077, 19.3561)
  line L183 (25.8077, 19.3561) -> (26.385, 18.3561)
  line L184 (26.385, 18.3561) -> (25.8077, 17.3561)
  line L185 (25.8077, 17.3561) -> (24.653, 17.3561)
  line L186 (24.653, 17.3561) -> (24.0756, 18.3561)
  line L187 (24.0756, 18.3561) -> (24.653, 19.3561)
  line L188 (30.3077, -13.5772) -> (30.885, -14.5772)
  line L189 (30.885, -14.5772) -> (30.3077, -15.5772)
  line L190 (30.3077, -15.5772) -> (29.153, -15.5772)
  line L191 (29.153, -15.5772) -> (28.5756, -14.5772)
  line L192 (28.5756, -14.5772) -> (29.153, -13.5772)
  line L193 (29.153, -13.5772) -> (30.3077, -13.5772)
  line L194 (26.3453, -10.755) -> (26.9227, -9.755)
  line L195 (26.9227, -9.755) -> (28.0774, -9.755)
  line L196 (28.0774, -9.755) -> (28.6547, -10.755)
  line L197 (28.6547, -10.755) -> (28.0774, -11.755)
  line L198 (28.0774, -11.755) -> (26.9227, -11.755)
  line L199 (26.9227, -11.755) -> (26.3453, -10.755)
  line L200 (30.3077, -11.0439) -> (30.885, -12.0439)
  line L201 (30.885, -12.0439) -> (30.3077, -13.0439)
  line L202 (30.3077, -13.0439) -> (29.153, -13.0439)
  line L203 (29.153, -13.0439) -> (28.5756, -12.0439)
  line L204 (28.5756, -12.0439) -> (29.153, -11.0439)
  line L205 (29.153, -11.0439) -> (30.3077, -11.0439)
  line L206 (26.3453, -8.2217) -> (26.9227, -7.2217)
  line L207 (26.9227, -7.2217) -> (28.0774, -7.2217)
  line L208 (28.0774, -7.2217) -> (28.6547, -8.2217)
  line L209 (28.6547, -8.2217) -> (28.0774, -9.2217)
  line L210 (28.0774, -9.2217) -> (26.9227, -9.2217)
  line L211 (26.9227, -9.2217) -> (26.3453, -8.2217)
  line L212 (21.8453, -10.755) -> (22.4227, -9.755)
  line L213 (22.4227, -9.755) -> (23.5774, -9.755)
  line L214 (23.5774, -9.755) -> (24.1547, -10.755)
  line L215 (24.1547, -10.755) -> (23.5774, -11.755)
  line L216 (23.5774, -11.755) -> (22.4227, -11.755)
  line L217 (22.4227, -11.755) -> (21.8453, -10.755)
  line L218 (30.3077, -16.1105) -> (30.885, -17.1105)
  line L219 (30.885, -17.1105) -> (30.3077, -18.1105)
  line L220 (30.3077, -18.1105) -> (29.153, -18.1105)
  line L221 (29.153, -18.1105) -> (28.5756, -17.1105)
  line L222 (28.5756, -17.1105) -> (29.153, -16.1105)
  line L223 (29.153, -16.1105) -> (30.3077, -16.1105)
  line L224 (30.3077, 9.2228) -> (30.885, 8.2228)
  line L225 (30.885, 8.2228) -> (30.3077, 7.2228)
  line L226 (30.3077, 7.2228) -> (29.153, 7.2228)
  line L227 (29.153, 7.2228) -> (28.5756, 8.2228)
  line L228 (28.5756, 8.2228) -> (29.153, 9.2228)
  line L229 (29.153, 9.2228) -> (30.3077, 9.2228)
  line L230 (25.8077, 14.2895) -> (26.385, 13.2895)
  line L231 (26.385, 13.2895) -> (25.8077, 12.2895)
  line L232 (25.8077, 12.2895) -> (24.653, 12.2895)
  line L233 (24.653, 12.2895) -> (24.0756, 13.2895)
  line L234 (24.0756, 13.2895) -> (24.653, 14.2895)
  line L235 (24.653, 14.2895) -> (25.8077, 14.2895)
  line L236 (30.3077, 14.2895) -> (30.885, 13.2895)
  line L237 (30.885, 13.2895) -> (30.3077, 12.2895)
  line L238 (30.3077, 12.2895) -> (29.153, 12.2895)
  line L239 (29.153, 12.2895) -> (28.5756, 13.2895)
  line L240 (28.5756, 13.2895) -> (29.153, 14.2895)
  line L241 (29.153, 14.2895) -> (30.3077, 14.2895)
  line L242 (30.3077, 11.7561) -> (30.885, 10.7561)
  line L243 (30.885, 10.7561) -> (30.3077, 9.7561)
  line L244 (30.3077, 9.7561) -> (29.153, 9.7561)
  line L245 (29.153, 9.7561) -> (28.5756, 10.7561)
  line L246 (28.5756, 10.7561) -> (29.153, 11.7561)
  line L247 (29.153, 11.7561) -> (30.3077, 11.7561)
  line L248 (25.8077, -8.5105) -> (26.385, -9.5105)
  line L249 (26.385, -9.5105) -> (25.8077, -10.5105)
  line L250 (25.8077, -10.5105) -> (24.653, -10.5105)
  line L251 (24.653, -10.5105) -> (24.0756, -9.5105)
  line L252 (24.0756, -9.5105) -> (24.653, -8.5105)
  line L253 (24.653, -8.5105) -> (25.8077, -8.5105)
  line L254 (26.3453, -15.8217) -> (26.9227, -14.8217)
  line L255 (26.9227, -14.8217) -> (28.0774, -14.8217)
  line L256 (28.0774, -14.8217) -> (28.6547, -15.8217)
  line L257 (28.6547, -15.8217) -> (28.0774, -16.8217)
  line L258 (28.0774, -16.8217) -> (26.9227, -16.8217)
  line L259 (26.9227, -16.8217) -> (26.3453, -15.8217)
  line L260 (26.3453, -18.355) -> (26.9227, -17.355)
  line L261 (26.9227, -17.355) -> (28.0774, -17.355)
  line L262 (28.0774, -17.355) -> (28.6547, -18.355)
  line L263 (28.6547, -18.355) -> (28.0774, -19.355)
  line L264 (28.0774, -19.355) -> (26.9227, -19.355)
  line L265 (26.9227, -19.355) -> (26.3453, -18.355)
  line L266 (21.8453, 9.5117) -> (22.4227, 10.5117)
  line L267 (22.4227, 10.5117) -> (23.5774, 10.5117)
  line L268 (23.5774, 10.5117) -> (24.1547, 9.5117)
  line L269 (24.1547, 9.5117) -> (23.5774, 8.5117)
  line L270 (23.5774, 8.5117) -> (22.4227, 8.5117)
  line L271 (22.4227, 8.5117) -> (21.8453, 9.5117)
  line L272 (26.3453, -13.2883) -> (26.9227, -12.2883)
  line L273 (26.9227, -12.2883) -> (28.0774, -12.2883)
  line L274 (28.0774, -12.2883) -> (28.6547, -13.2883)
  line L275 (28.6547, -13.2883) -> (28.0774, -14.2883)
  line L276 (28.0774, -14.2883) -> (26.9227, -14.2883)
  line L277 (26.9227, -14.2883) -> (26.3453, -13.2883)
  line L278 (25.8077, -16.1105) -> (26.385, -17.1105)
  line L279 (26.385, -17.1105) -> (25.8077, -18.1105)
  line L280 (25.8077, -18.1105) -> (24.653, -18.1105)
  line L281 (24.653, -18.1105) -> (24.0756, -17.1105)
  line L282 (24.0756, -17.1105) -> (24.653, -16.1105)
  line L283 (24.653, -16.1105) -> (25.8077, -16.1105)
  line L284 (30.3077, 16.8228) -> (30.885, 15.8228)
  line L285 (30.885, 15.8228) -> (30.3077, 14.8228)
  line L286 (30.3077, 14.8228) -> (29.153, 14.8228)
  line L287 (29.153, 14.8228) -> (28.5756, 15.8228)
  line L288 (28.5756, 15.8228) -> (29.153, 16.8228)
  line L289 (29.153, 16.8228) -> (30.3077, 16.8228)
  line L290 (30.3077, -3.4439) -> (30.885, -4.4439)
  line L291 (30.885, -4.4439) -> (30.3077, -5.4439)
  line L292 (30.3077, -5.4439) -> (29.153, -5.4439)
  line L293 (29.153, -5.4439) -> (28.5756, -4.4439)
  line L294 (28.5756, -4.4439) -> (29.153, -3.4439)
  line L295 (29.153, -3.4439) -> (30.3077, -3.4439)
  line L296 (25.8077, -13.5772) -> (26.385, -14.5772)
  line L297 (26.385, -14.5772) -> (25.8077, -15.5772)
  line L298 (25.8077, -15.5772) -> (24.653, -15.5772)
  line L299 (24.653, -15.5772) -> (24.0756, -14.5772)
  line L300 (24.0756, -14.5772) -> (24.653, -13.5772)
  line L301 (24.653, -13.5772) -> (25.8077, -13.5772)
  line L302 (26.3453, 14.5783) -> (26.9227, 15.5783)
  line L303 (26.9227, 15.5783) -> (28.0774, 15.5783)
  line L304 (28.0774, 15.5783) -> (28.6547, 14.5783)
  line L305 (28.6547, 14.5783) -> (28.0774, 13.5783)
  line L306 (28.0774, 13.5783) -> (26.9227, 13.5783)
  line L307 (26.9227, 13.5783) -> (26.3453, 14.5783)
  line L308 (21.8453, -5.6883) -> (22.4227, -4.6883)
  line L309 (22.4227, -4.6883) -> (23.5774, -4.6883)
  line L310 (23.5774, -4.6883) -> (24.1547, -5.6883)
  line L311 (24.1547, -5.6883) -> (23.5774, -6.6883)
  line L312 (23.5774, -6.6883) -> (22.4227, -6.6883)
  line L313 (22.4227, -6.6883) -> (21.8453, -5.6883)
  line L314 (25.8077, 11.7561) -> (26.385, 10.7561)
  line L315 (26.385, 10.7561) -> (25.8077, 9.7561)
  line L316 (25.8077, 9.7561) -> (24.653, 9.7561)
  line L317 (24.653, 9.7561) -> (24.0756, 10.7561)
  line L318 (24.0756, 10.7561) -> (24.653, 11.7561)
  line L319 (24.653, 11.7561) -> (25.8077, 11.7561)
  line L320 (21.8453, 12.045) -> (22.4227, 13.045)
  line L321 (22.4227, 13.045) -> (23.5774, 13.045)
  line L322 (23.5774, 13.045) -> (24.1547, 12.045)
  line L323 (24.1547, 12.045) -> (23.5774, 11.045)
  line L324 (23.5774, 11.045) -> (22.4227, 11.045)
  line L325 (22.4227, 11.045) -> (21.8453, 12.045)
  line L326 (30.3077, -5.9772) -> (30.885, -6.9772)
  line L327 (30.885, -6.9772) -> (30.3077, -7.9772)
  line L328 (30.3077, -7.9772) -> (29.153, -7.9772)
  line L329 (29.153, -7.9772) -> (28.5756, -6.9772)
  line L330 (28.5756, -6.9772) -> (29.153, -5.9772)
  line L331 (29.153, -5.9772) -> (30.3077, -5.9772)
  line L332 (21.8453, 14.5783) -> (22.4227, 15.5783)
  line L333 (22.4227, 15.5783) -> (23.5774, 15.5783)
  line L334 (23.5774, 15.5783) -> (24.1547, 14.5783)
  line L335 (24.1547, 14.5783) -> (23.5774, 13.5783)
  line L336 (23.5774, 13.5783) -> (22.4227, 13.5783)
  line L337 (22.4227, 13.5783) -> (21.8453, 14.5783)
  line L338 (21.8453, -13.2883) -> (22.4227, -12.2883)
  line L339 (22.4227, -12.2883) -> (23.5774, -12.2883)
  line L340 (23.5774, -12.2883) -> (24.1547, -13.2883)
  line L341 (24.1547, -13.2883) -> (23.5774, -14.2883)
  line L342 (23.5774, -14.2883) -> (22.4227, -14.2883)
  line L343 (22.4227, -14.2883) -> (21.8453, -13.2883)
  line L344 (26.3453, -5.6883) -> (26.9227, -4.6883)
  line L345 (26.9227, -4.6883) -> (28.0774, -4.6883)
  line L346 (28.0774, -4.6883) -> (28.6547, -5.6883)
  line L347 (28.6547, -5.6883) -> (28.0774, -6.6883)
  line L348 (28.0774, -6.6883) -> (26.9227, -6.6883)
  line L349 (26.9227, -6.6883) -> (26.3453, -5.6883)
  line L350 (30.3077, -8.5105) -> (30.885, -9.5105)
  line L351 (30.885, -9.5105) -> (30.3077, -10.5105)
  line L352 (30.3077, -10.5105) -> (29.153, -10.5105)
  line L353 (29.153, -10.5105) -> (28.5756, -9.5105)
  line L354 (28.5756, -9.5105) -> (29.153, -8.5105)
  line L355 (29.153, -8.5105) -> (30.3077, -8.5105)
  line L356 (21.8453, -8.2217) -> (22.4227, -7.2217)
  line L357 (22.4227, -7.2217) -> (23.5774, -7.2217)
  line L358 (23.5774, -7.2217) -> (24.1547, -8.2217)
  line L359 (24.1547, -8.2217) -> (23.5774, -9.2217)
  line L360 (23.5774, -9.2217) -> (22.4227, -9.2217)
  line L361 (22.4227, -9.2217) -> (21.8453, -8.2217)
  line L362 (25.8077, 6.6895) -> (26.385, 5.6895)
  line L363 (26.385, 5.6895) -> (25.8077, 4.6895)
  line L364 (25.8077, 4.6895) -> (24.653, 4.6895)
  line L365 (24.653, 4.6895) -> (24.0756, 5.6895)
  line L366 (24.0756, 5.6895) -> (24.653, 6.6895)
  line L367 (24.653, 6.6895) -> (25.8077, 6.6895)
  line L368 (26.3453, 9.5117) -> (26.9227, 10.5117)
  line L369 (26.9227, 10.5117) -> (28.0774, 10.5117)
  line L370 (28.0774, 10.5117) -> (28.6547, 9.5117)
  line L371 (28.6547, 9.5117) -> (28.0774, 8.5117)
  line L372 (28.0774, 8.5117) -> (26.9227, 8.5117)
  line L373 (26.9227, 8.5117) -> (26.3453, 9.5117)
  line L374 (25.8077, 4.1561) -> (26.385, 3.1561)
  line L375 (26.385, 3.1561) -> (25.8077, 2.1561)
  line L376 (25.8077, 2.1561) -> (24.653, 2.1561)
  line L377 (24.653, 2.1561) -> (24.0756, 3.1561)
  line L378 (24.0756, 3.1561) -> (24.653, 4.1561)
  line L379 (24.653, 4.1561) -> (25.8077, 4.1561)
  line L380 (25.8077, -18.6439) -> (26.385, -19.6439)
  line L381 (26.385, -19.6439) -> (25.8077, -20.6439)
  line L382 (25.8077, -20.6439) -> (24.653, -20.6439)
  line L383 (24.653, -20.6439) -> (24.0756, -19.6439)
  line L384 (24.0756, -19.6439) -> (24.653, -18.6439)
  line L385 (24.653, -18.6439) -> (25.8077, -18.6439)
  line L386 (21.8453, -18.355) -> (22.4227, -17.355)
  line L387 (22.4227, -17.355) -> (23.5774, -17.355)
  line L388 (23.5774, -17.355) -> (24.1547, -18.355)
  line L389 (24.1547, -18.355) -> (23.5774, -19.355)
  line L390 (23.5774, -19.355) -> (22.4227, -19.355)
  line L391 (22.4227, -19.355) -> (21.8453, -18.355)
  line L392 (21.8453, 4.445) -> (22.4227, 5.445)
  line L393 (22.4227, 5.445) -> (23.5774, 5.445)
  line L394 (23.5774, 5.445) -> (24.1547, 4.445)
  line L395 (24.1547, 4.445) -> (23.5774, 3.445)
  line L396 (23.5774, 3.445) -> (22.4227, 3.445)
  line L397 (22.4227, 3.445) -> (21.8453, 4.445)
  line L398 (26.3453, 17.1117) -> (26.9227, 18.1117)
  line L399 (26.9227, 18.1117) -> (28.0774, 18.1117)
  line L400 (28.0774, 18.1117) -> (28.6547, 17.1117)
  line L401 (28.6547, 17.1117) -> (28.0774, 16.1117)
  line L402 (28.0774, 16.1117) -> (26.9227, 16.1117)
  line L403 (26.9227, 16.1117) -> (26.3453, 17.1117)
  dimension "d41" = 23
  dimension "d42" = 5.5
  dimension "d43" = 31
  dimension "d44" = 15
  dimension "d45" = 2
  dimension "d46" = 4
  dimension "d47" = 4.5
  dimension "d48" = 18
  dimension "d49" = 8.75
  dimension "d50" = 3
  dimension "d51" = 16
  dimension "d52" = 1
  constraint horizontal L4
  constraint vertical L5
  constraint horizontal L6
  constraint vertical L7
  constraint coincident L2 L4.start
  constraint horizontal L8
  constraint vertical L9
  constraint horizontal L10
  constraint vertical L11
  constraint coincident L6 L8.start
  constraint horizontal L12
  constraint vertical L13
  constraint horizontal L14
  constraint vertical L15
  constraint coincident L1 L12.start
  constraint horizontal L16
  constraint vertical L17
  constraint horizontal L18
  constraint vertical L19
  constraint coincident L13 L16.start
  measures "d41" distance of L4.start L4.end
  measures "d42" distance of L4.start L6.end
  measures "d43" distance of L3 L7
  measures "d44" distance of L8.start L8.end
  measures "d45" distance of L8.start L10.end
  measures "d46" distance of L7 L11
  measures "d47" distance of L12.start L12.end
  measures "d48" distance of L12.start L14.end
  measures "d49" distance of L2 L12
  measures "d50" distance of L16.start L16.end
  measures "d51" distance of L16.start L18.end
  measures "d52" distance of L12 L16
extrude "Extrude2" add sketch "Sketch2" along normal blind 27 contours L1 L12 L13 L14 L15 L19
extrude "Extrude3" add sketch "Sketch2" along normal blind 27 contours L13 L16 L17 L18 L19
extrude "Extrude4" add sketch "Sketch2" along normal blind 30.5 contours L2 L4 L5 L6 L7 L8
extrude "Extrude5" add sketch "Sketch2" along normal blind 34 contours L6 L8 L9 L10 L11
